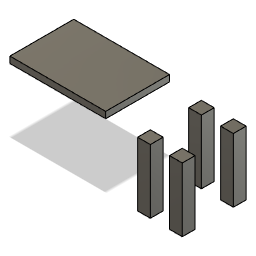
02-joint-rigid (Autodesk Fusion 360 design; units mm, degrees)
Autodesk Fusion 360 part; units mm, degrees
sketch "スケッチ1" plane through (0, 0, 0) normal (0, 1, 0) x (1, 0, 0)
  line L0 (0, 0) -> (75, 0)
  line L1 (75, 0) -> (75, 50)
  line L2 (75, 50) -> (0, 50)
  line L3 (0, 50) -> (0, 0)
  line L4 (100, 10) -> (110, 10)
  line L5 (110, 10) -> (110, 0)
  line L6 (110, 0) -> (100, 0)
  line L7 (100, 0) -> (100, 10)
  constraint horizontal L0
  constraint vertical L1
  constraint horizontal L2
  constraint vertical L3
  constraint coincident L0.start L3.end
  constraint horizontal L4
  constraint vertical L5
  constraint horizontal L6
  constraint vertical L7
extrude "押し出し1" add sketch "スケッチ1" along normal blind 5 from surface at 50 contours L0 L1 L2 L3 makes body 1 in component "天板"
extrude "押し出し1'" add sketch "スケッチ1" along normal blind 50 separate body contours L4 L5 L6 L7 makes body 2 in component "足"
component "天板" placed x (1, 0, 0) y (0, 1, 0) z (0, 0, 1) at (0, 0, 0)
component "足" placed x (1, 0, 0) y (0, 1, 0) z (0, 0, 1) at (0, 0, 0)
component "足" placed x (1, 0, 0) y (0, 1, 0) z (0, 0, 1) at (25, 0, 0)
component "足" placed x (1, 0, 0) y (0, 1, 0) z (0, 0, 1) at (0, 0, -40)
component "足" placed x (1, 0, 0) y (0, 1, 0) z (0, 0, 1) at (25, 0, -40)
